vSlot Bolt Head 30mm M6 July 13 (Autodesk Fusion 360 design; units mm, degrees)
Autodesk Fusion 360 part; units mm, degrees
sketch "Sketch1" plane through (0, 0, 0) normal (0, 0, 1) x (1, 0, 0)
  line L0 (-3.5, 0) -> (3.5, 0)
  line L1 (3.5, 0) -> (7.75, 4.25)
  line L2 (7.75, 4.25) -> (7.75, 6)
  line L3 (-3.5, 0) -> (-7.75, 4.25)
  line L4 (-7.75, 4.25) -> (-7.75, 6)
  line L5 (-7.75, 6) -> (7.75, 6)
  dimension "d1" = 7
  dimension "d2" = 6
  dimension "d3" = 45
  dimension "d4" = 45
  dimension "d5" = 15.5
  measures "d1" distance of L0.start L0.end
  measures "d2" distance of L0.end L2.end
  measures "d3" angle of L0 L1
  measures "d4" angle of L0 L3
  measures "d5" distance of L2 L4
extrude "Extrude1" add sketch "Sketch1" along normal blind 15
sketch "Sketch2" plane through (0, 0, 0) normal (0, -1, 0) x (1, 0, 0)
  line L0 (-3.5, 0) -> (3.5, 0)
  line L1 (3.5, 0) -> (3.5, 15)
  line L2 (3.5, 15) -> (-3.5, 15)
  line L3 (-3.5, 15) -> (-3.5, 0)
  line L4 (0, 13.389) -> (-5.1, 10.4445)
  line L5 (-5.1, 10.4445) -> (-5.1, 4.5555)
  line L6 (-5.1, 4.5555) -> (0, 1.611)
  line L7 (0, 1.611) -> (5.1, 4.5555)
  line L8 (5.1, 4.5555) -> (5.1, 10.4445)
  line L9 (5.1, 10.4445) -> (0, 13.389)
  point P0 (0, 7.5)
  point P1 (3.5, 7.5)
  dimension "d8" = 10.2
  measures "d8" distance of L6 L9
extrude "Extrude2" cut sketch "Sketch2" against normal blind 4 contours L3 L4 L5 L6 | L1 L3 L4 L6 L7 L9 | L1 L7 L8 L9
sketch "Sketch3" plane through (0, 4, 0) normal (0, -1, 0) x (1, 0, 0)
  line L0 (5.1, 10.4445) -> (0, 13.389)
  line L1 (0, 13.389) -> (-5.1, 10.4445)
  line L2 (-5.1, 10.4445) -> (-5.1, 4.5555)
  line L3 (-5.1, 4.5555) -> (0, 1.611)
  line L4 (0, 1.611) -> (5.1, 4.5555)
  line L5 (5.1, 4.5555) -> (5.1, 10.4445)
  line L6 (0, 13.389) -> (0, 1.611) construction
  circle A0 centre (0, 7.5) radius 3.125
  point P0 (0, 1.611)
  point P1 (0, 13.389)
  dimension "d11" = 6.25
  measures "d11" diameter of A0
extrude "Extrude3" cut sketch "Sketch3" against normal through all contours A0
fillet "Fillet1" radius 1 6 edges at (3.5, 0, 1.8159) (3.5, 0, 13.1841) (-3.5, 0, 13.1841) (-3.5, 0, 1.8159) (-5.1, 1.6, 7.5) (5.1, 1.6, 7.5)
